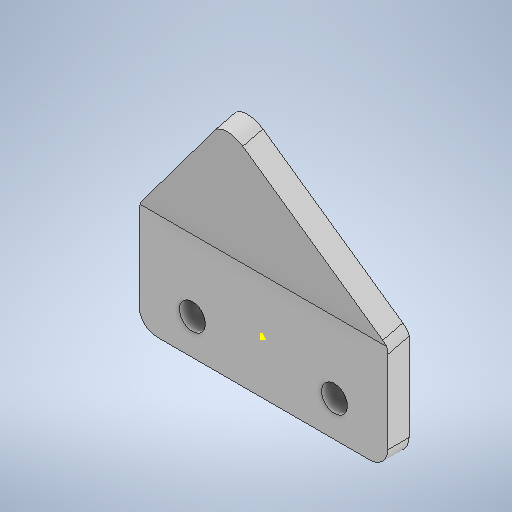
# Autodesk Inventor part: Hook
Saved by Autodesk Inventor 2025.1 (Build 291241020, 241B)
## iProperties
Created: 2024-11-21
Part Number: Hook
Material: Generic
Document SubType Name: Modeling
Designer: AtuStem
Density: 1 g/cm^3
Appearance: Default
Author: AtuStem
Autodesk Inventor part; units mm, degrees
ref_plane "YZ Plane" through (0, 0, 0) normal (1, 0, 0) x (0, 1, 0)
ref_plane "XZ Plane" through (0, 0, 0) normal (0, 1, 0) x (-1, 0, 0)
ref_plane "XY Plane" through (0, 0, 0) normal (0, 0, 1) x (1, 0, 0)
sketch "Sketch1" plane through (0, 0, 0) normal (0, 0, 1) x (1, 0, 0)
  line L0 (-22.225, 9.525) -> (22.225, 9.525)
  line L1 (22.225, 9.525) -> (22.225, -9.525)
  line L2 (22.225, -9.525) -> (-22.225, -9.525)
  line L3 (-22.225, -9.525) -> (-22.225, 9.525)
  line L4 (-22.225, 9.525) -> (22.225, -9.525) construction
  line L5 (22.225, 9.525) -> (-22.225, -9.525) construction
  point P0 (0, 0)
  dimension "d0" = 44.45
  dimension "d18" = 19.05
  constraints: 12 end point, 2 midpoint, 2 parallel, 1 horizontal, 1 perpendicular
  measures "d0" distance of L1.end L2.end
  measures "d18" distance of L2.end L0.start
extrude "Extrusion1" add sketch "Sketch1" along normal blind 3.81
sketch "Sketch2" plane through (22.225, -9.525, 0) normal (1, 0, 0) x (0, 0, -1)
  line L0 (0, 0) -> (0, 19.05) projected
  line L1 (0, 19.05) -> (-7.1849, 47.3626)
  line L2 (-3.81, 19.05) -> (0, 19.05)
  line L3 (-3.81, 19.05) -> (-10.7644, 46.4542)
  line L4 (-10.7644, 46.4542) -> (-7.1849, 47.3626)
  point P0 (0, 9.525)
  dimension "d3" = 29.21
  constraints: 8 end point, 2 perpendicular
  measures "d3" distance of L0.end L1.end
extrude "Extrusion2" add sketch "Sketch2" against normal blind 44.45
sketch "Sketch3" plane through (-22.225, 36.9292, 10.7644) normal (0, -0.2459747, 0.9692762) x (1, 0, 0)
  line L0 (0, 0) -> (0, -29.21) projected
  line L1 (44.45, 0) -> (0, 0) projected
  line L2 (44.45, -29.21) -> (44.45, 0) projected
  line L3 (22.225, 0) -> (44.45, 0)
  line L4 (44.45, 0) -> (44.45, -14.605)
  line L5 (22.225, 0) -> (0, 0)
  line L6 (0, 0) -> (0, -14.605)
  line L7 (44.45, -28.2728) -> (0, -28.2728) projected
  line L8 (0, -28.2728) -> (44.45, -28.2728)
  line L9 (44.45, -28.2728) -> (0, -28.2728)
  line L10 (0, -28.2728) -> (22.225, 0)
  line L11 (22.225, 0) -> (44.45, -28.2728)
  point P0 (22.225, -38.4424)
  constraints: 16 end point, 3 collinear, 3 midpoint, 2 perpendicular, 1 horizontal, 1 point on line
extrude "Extrusion3" cut sketch "Sketch3" against normal blind 72.39 contours L1 L10 L0 | L1 L2 L11
sketch "Sketch5" plane through (0, 0, 3.81) normal (0, 0, 1) x (1, 0, 0)
  line L0 (-22.225, -9.525) -> (22.225, -9.525) projected
  line L1 (-22.225, -9.525) -> (-22.225, -3.175)
  line L2 (-22.225, 9.525) -> (-22.225, -9.525) projected
  line L3 (-22.225, -3.175) -> (22.225, -3.175)
  line L4 (22.225, -3.175) -> (22.225, -9.525)
  line L5 (-22.225, -3.175) -> (0, -3.175)
  line L6 (-11.1125, -3.175) -> (14.2875, -3.175)
  line L7 (-22.225, -3.175) -> (-12.7, -3.175)
  line L8 (-12.7, -3.175) -> (12.7, -3.175)
  line L9 (12.7, -3.175) -> (22.225, -3.175)
  circle A0 centre (-12.7, -3.175) radius 2.3241
  circle A1 centre (12.7, -3.175) radius 2.3241
  point P0 (0, 0)
  dimension "d11" = 6.35
  dimension "d23" = 9.525
  dimension "d24" = 25.4
  dimension "d25" = 4.6482
  dimension "d26" = 4.6482
  constraints: 16 end point, 4 point on line, 2 centre point, 2 coincident, 2 midpoint, 1 collinear, 1 horizontal, 1 perpendicular
  measures "d11" distance of L0.start L1.end
  measures "d23" distance of L1.end L7.end
  measures "d24" distance of L7.end L8.end
  measures "d25" diameter of A0
  measures "d26" diameter of A1
extrude "Extrusion4" cut sketch "Sketch5" against normal blind 50.8 contours A0 L3 | L3 A0 | A1 L3 | L3 A1
fillet "Fillet1" radius 3.175 1 edges at (0, 37.3834, 8.9747)
fillet "Fillet2" radius 3.175 4 edges at (22.225, -9.525, 1.905) (-22.225, -9.525, 1.905) (-22.225, 9.9792, 2.0203) (22.225, 9.9792, 2.0203)
sketch "Sketch6" plane through (0, 0, 3.81) normal (0, 0, 1) x (1, 0, 0)
  point P0 (0, 0)
body "Solid1"
